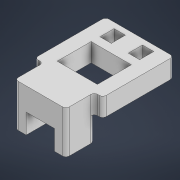
# Autodesk Inventor part: QRholder-bottom
Saved by Autodesk Inventor 2022 (Build 260153000, 153)
## iProperties
Created: 2023-05-02
Part Number: QRholder-bottom
Material: Všeobecné
Document SubType Name: Modeling
Designer: tada
Density: 1 g/cm^3
Appearance: Výchozí
Author: tada
Autodesk Inventor part; units mm, degrees
ref_plane "YZ Plane" through (0, 0, 0) normal (1, 0, 0) x (0, 1, 0)
ref_plane "XZ Plane" through (0, 0, 0) normal (0, 1, 0) x (-1, 0, 0)
ref_plane "XY Plane" through (0, 0, 0) normal (0, 0, 1) x (1, 0, 0)
sketch "Náčrt1" plane through (0, 0, 0) normal (0, 0, 1) x (1, 0, 0)
  line L0 (-9, 0) -> (-5, 0)
  line L1 (-5, 0) -> (-5, 7)
  line L2 (-5, 7) -> (5, 7)
  line L3 (5, 7) -> (5, 0)
  line L4 (9, 0) -> (9, 15)
  line L5 (9, 15) -> (-9, 15)
  line L6 (-9, 15) -> (-9, 0)
  line L7 (5, 0) -> (9, 0)
  point P0 (0, 0)
  dimension "d0" = 10
  dimension "d1" = 4
  dimension "d2" = 4
  dimension "d3" = 5
  dimension "d4" = 7
  dimension "d5" = 7
  dimension "d8" = 8
  constraints: 16 end point, 5 perpendicular, 2 horizontal, 1 point on line
  measures "d0" distance between parallel lines of L3 L1
  measures "d1" distance between parallel lines of L4 L3
  measures "d2" distance between parallel lines of L6 L1
  measures "d3" distance from line of L3 point (0, 0)
  measures "d4" distance from line of L2 point (0, 0)
  measures "d5" distance between parallel lines of L2 L7
  measures "d8" distance between parallel lines of L5 L2
extrude "Vysunutí1" add sketch "Náčrt1" along normal blind 10
sketch "Náčrt2" plane through (0, 0, 0) normal (0, 0, -1) x (-1, 0, 0)
  line L0 (5, 7) -> (-5, 7) projected
  line L1 (-12, 15) -> (12, 15)
  line L2 (12, 15) -> (12, 8.5)
  line L3 (12, 8.5) -> (-12, 8.5)
  line L4 (-12, 8.5) -> (-12, 15)
  line L5 (-9, 15) -> (9, 15) projected
  line L6 (-9, 0) -> (-9, 15) projected
  line L7 (9, 15) -> (9, 0) projected
  point P0 (0, 0)
  dimension "d19" = 1.5
  dimension "d20" = 3
  dimension "d21" = 3
  constraints: 8 end point, 2 collinear, 2 parallel, 1 horizontal, 1 perpendicular
  measures "d19" distance between parallel lines of L3 L0
  measures "d20" distance between parallel lines of L4 L6
  measures "d21" distance between parallel lines of L7 L2
extrude "Vysunutí4" add sketch "Náčrt2" along normal blind 15
sketch "Náčrt4" plane through (-9, 15, 10) normal (0, 1, 0) x (1, 0, 0)
  line L0 (21, 25) -> (-3, 25) projected
  line L1 (1.9, 25) -> (16.1, 25)
  line L2 (16.1, 25) -> (16.1, 13)
  line L3 (16.1, 13) -> (1.9, 13)
  line L4 (1.9, 13) -> (1.9, 25)
  line L5 (21, 10) -> (21, 25) projected
  line L6 (-3, 10) -> (-3, 25) projected
  point P0 (9, 10)
  dimension "d24" = 12
  dimension "d25" = 4.9
  dimension "d26" = 4.9
  constraints: 8 end point, 2 parallel, 1 horizontal, 1 perpendicular, 1 point on line
  measures "d24" distance between parallel lines of L3 L0
  measures "d25" distance between parallel lines of L5 L2
  measures "d26" distance between parallel lines of L6 L4
extrude "Vysunutí5" cut sketch "Náčrt4" against normal blind 15
sketch "Náčrt5" plane through (0, 0, -15) normal (0, 0, -1) x (-1, 0, 0)
  line L0 (-7.1, 15) -> (-12, 15) projected
  line L1 (12, 8.5) -> (12, 15) projected
  line L2 (-12, 15) -> (12, 15)
  line L3 (12, 15) -> (12, 8.5)
  line L4 (12, 8.5) -> (-12, 8.5)
  line L5 (-12, 8.5) -> (-12, 15)
  point P0 (0, 0)
  constraints: 8 end point, 2 parallel, 1 horizontal, 1 perpendicular
extrude "Vysunutí6" add sketch "Náčrt5" along normal blind 10
sketch "Náčrt6" plane through (-9, 15, 10) normal (0, 1, 0) x (1, 0, 0)
  line L0 (2, 28) -> (6, 28)
  line L1 (6, 28) -> (6, 33)
  line L2 (6, 33) -> (2, 33)
  line L3 (2, 33) -> (2, 28)
  line L4 (12, 28) -> (16, 28)
  line L5 (16, 28) -> (16, 33)
  line L6 (16, 33) -> (12, 33)
  line L7 (12, 33) -> (12, 28)
  line L8 (-3, 10) -> (-3, 35) projected
  line L9 (21, 10) -> (21, 35) projected
  line L10 (1.9, 25) -> (16.1, 25) projected
  line L11 (-3, 35) -> (21, 35) projected
  point P0 (9, 10)
  dimension "d33" = 3
  dimension "d34" = 3
  dimension "d35" = 2
  dimension "d36" = 2
  dimension "d38" = 4
  dimension "d39" = 4
  dimension "d45" = 6
  dimension "d46" = 5
  dimension "d47" = 5
  constraints: 16 end point, 4 parallel, 2 horizontal, 2 perpendicular
  measures "d33" distance between parallel lines of L10 L0
  measures "d34" distance between parallel lines of L10 L4
  measures "d35" distance between parallel lines of L11 L2
  measures "d36" distance between parallel lines of L11 L6
  measures "d38" distance between parallel lines of L3 L1
  measures "d39" distance between parallel lines of L7 L5
  measures "d45" distance between parallel lines of L7 L1
  measures "d46" distance between parallel lines of L8 L3
  measures "d47" distance between parallel lines of L9 L5
extrude "Vysunutí7" cut sketch "Náčrt6" against normal blind 10
fillet "Zaoblení2" radius 1.2 10 edges at (-9, 7.5, 10) (-9, 4.25, 0) (9, 4.25, 0) (9, 7.5, 10) (9, 11.75, 0) (12, 11.75, 0) (-9, 11.75, 0) (-12, 11.75, 0) (-12, 11.75, -25) (12, 11.75, -25)
equation "\"d2\" = d1"
equation "\"d3\" = 0.5 * d0"
equation "\"d5\" = d4"
equation "\"d21\" = d20"
equation "\"d26\" = d25"
equation "\"d34\" = d33"
equation "\"d36\" = d35"
equation "\"d39\" = d38"
